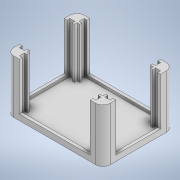
# Autodesk Inventor part: small_bottom
Saved by Autodesk Inventor 2021 (Build 250183000, 183)
## iProperties
Created: 2021-08-22
Part Number: small_bottom
Material: Generisch
Document SubType Name: Modeling
Designer: Tilman
Density: 1 g/cm^3
Appearance: Vorgabe
Author: Tilman
Autodesk Inventor part; units mm, degrees
ref_plane "YZ Plane" through (0, 0, 0) normal (1, 0, 0) x (0, 1, 0)
ref_plane "XZ Plane" through (0, 0, 0) normal (0, 1, 0) x (-1, 0, 0)
ref_plane "XY Plane" through (0, 0, 0) normal (0, 0, 1) x (1, 0, 0)
sketch "Skizze1" plane through (0, 0, 0) normal (0, 1, 0) x (-1, 0, 0)
  line L0 (-5, 0) -> (-62, 0)
  line L1 (-67, -5) -> (-67, -44)
  line L2 (-62, -49) -> (-5, -49)
  line L3 (0, -44) -> (0, -5)
  arc A0 (0, -5) -> (-5, 0) centre (-5, -5) ccw
  arc A1 (-62, 0) -> (-67, -5) centre (-62, -5) ccw
  arc A2 (-67, -44) -> (-62, -49) centre (-62, -44) ccw
  arc A3 (-5, -49) -> (0, -44) centre (-5, -44) ccw
  point P0 (0, 0)
  point P1 (-67, -49)
  point P2 (-67, 0)
  point P3 (0, -49)
  dimension "d0" = 67
  dimension "d1" = 49
  dimension "d2" = 5
  constraints: 8 end point, 8 point on circle, 8 point on line, 8 tangent, 4 centre point, 3 equal radius, 2 parallel, 1 horizontal, 1 perpendicular
  measures "d0" distance of point (-67, -49) point (0, -49)
  measures "d1" distance of point (-67, 0) point (-67, -49)
  measures "d2" radius of A0
extrude "Extrusion1" add sketch "Skizze1" along normal blind 2
sketch "Skizze2" plane through (0, 2, 0) normal (0, 1, 0) x (1, 0, 0)
  arc A0 (62, 0) -> (67, 5) centre (62, 5) ccw projected
  line L0 (67, 5) -> (67, 44) projected
  arc A1 (67, 44) -> (62, 49) centre (62, 44) ccw projected
  line L1 (62, 49) -> (5, 49) projected
  arc A2 (5, 49) -> (0, 44) centre (5, 44) ccw projected
  line L2 (0, 44) -> (0, 5) projected
  arc A3 (0, 5) -> (5, 0) centre (5, 5) ccw projected
  line L3 (5, 0) -> (62, 0) projected
  line L4 (6.9142, 5.5) -> (60.0858, 5.5)
  line L5 (60.0858, 5.5) -> (60.0858, 2)
  line L6 (60.0858, 2) -> (6.9142, 2)
  line L7 (6.9142, 2) -> (6.9142, 5.5)
  line L8 (61.5, 6.9142) -> (65, 6.9142)
  line L9 (65, 6.9142) -> (65, 42.0858)
  line L10 (65, 42.0858) -> (61.5, 42.0858)
  line L11 (61.5, 42.0858) -> (61.5, 6.9142)
  line L12 (60.0858, 47) -> (6.9142, 47)
  line L13 (6.9142, 47) -> (6.9142, 43.5)
  line L14 (6.9142, 43.5) -> (60.0858, 43.5)
  line L15 (60.0858, 43.5) -> (60.0858, 47)
  line L16 (2, 42.0858) -> (5.5, 42.0858)
  line L17 (5.5, 42.0858) -> (5.5, 6.9142)
  line L18 (5.5, 6.9142) -> (2, 6.9142)
  line L19 (2, 6.9142) -> (2, 42.0858)
  line L20 (33.5, 47) -> (33.5, 49) construction
  line L21 (65, 24.5) -> (67, 24.5) construction
  line L22 (62, 49) -> (5, 49) construction
  line L23 (33.5, 2) -> (33.5, 0) construction
  line L24 (5, 0) -> (62, 0) construction
  line L25 (2, 24.5) -> (0, 24.5) construction
  line L26 (0, 44) -> (0, 5) construction
  line L27 (5.5, 40.0858) -> (7, 40.0858)
  line L28 (7, 40.0858) -> (7, 42)
  line L29 (7, 42) -> (8.9142, 42)
  line L30 (8.9142, 42) -> (8.9142, 43.5)
  line L31 (61.5, 40.0858) -> (60, 40.0858)
  line L32 (60, 40.0858) -> (60, 42)
  line L33 (60, 42) -> (58.0858, 42)
  line L34 (58.0858, 42) -> (58.0858, 43.5)
  line L35 (61.5, 8.9142) -> (60, 8.9142)
  line L36 (60, 8.9142) -> (60, 7)
  line L37 (60, 7) -> (58.0858, 7)
  line L38 (58.0858, 7) -> (58.0858, 5.5)
  line L39 (8.9142, 5.5) -> (8.9142, 7)
  line L40 (8.9142, 7) -> (7, 7)
  line L41 (7, 7) -> (7, 8.9142)
  line L42 (7, 8.9142) -> (5.5, 8.9142)
  line L43 (2, 40.0858) -> (0, 40.0858)
  line L44 (65, 40.0858) -> (67, 40.0858)
  line L45 (65, 8.9142) -> (67, 8.9142)
  line L46 (58.0858, 2) -> (58.0858, 0)
  line L47 (8.9142, 2) -> (8.9142, 0)
  line L48 (2, 8.9142) -> (0, 8.9142)
  line L49 (8.9142, 47) -> (8.9142, 49)
  line L50 (58.0858, 47) -> (58.0858, 49)
  point P0 (0, 0)
  point P1 (58.0858, 0)
  point P2 (8.9142, 0)
  dimension "d5" = 3.5
  dimension "d6" = 2
  dimension "d7" = 35
  dimension "d9" = 2
  dimension "d10" = 2
  dimension "d11" = 2
  constraints: 88 end point, 30 point on line, 25 perpendicular, 20 equal length, 10 parallel, 8 midpoint, 6 horizontal alignment, 6 vertical alignment, 5 horizontal, 1 vertical
  measures "d5" distance of L12.end L13.end
  measures "d6" distance of L20.start L20.end
  measures "d7" distance between parallel lines of L40 L29
  measures "d9" distance between parallel lines of L18 L42
  measures "d10" distance between parallel lines of L7 L39
  measures "d11" distance of L17.end L4.start
extrude "Extrusion2" add sketch "Skizze2" along normal blind 2 contours L3 L47 L6 L46 | L45 L9 L44 L0 | L2 L43 L19 L48 | L50 L12 L49 L1
extrude "Extrusion3" add sketch "Skizze2" along normal blind 35 contours L3 L46 L6 L5 L4 L38 L37 L36 L35 L11 L8 L9 L45 L0 A0 | L3 A3 L2 L48 L19 L18 L17 L42 L41 L40 L39 L4 L7 L6 L47 | L44 L9 L10 L11 L31 L32 L33 L34 L14 L15 L12 L50 L1 A1 L0 | L2 A2 L1 L49 L12 L13 L14 L30 L29 L28 L27 L17 L16 L19 L43
equation "\"d10\" = d9"
